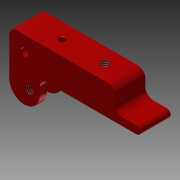
# Autodesk Inventor part: extruder_lever
Saved by Autodesk Inventor 2013 (Build 170138000, 138)
## iProperties
Created: 2015-02-21
Part Number: extruder_lever
Material: 一般
Document SubType Name: Modeling
Designer: Noa Izumi
Density: 1 g/cm^3
Author: Noa Izumi
Autodesk Inventor part; units mm, degrees
ref_plane "YZ Plane" through (0, 0, 0) normal (1, 0, 0) x (0, 1, 0)
ref_plane "XZ Plane" through (0, 0, 0) normal (0, 1, 0) x (-1, 0, 0)
ref_plane "XY Plane" through (0, 0, 0) normal (0, 0, 1) x (1, 0, 0)
sketch "草圖1" plane through (0, 0, 0) normal (0, 1, 0) x (-1, 0, 0)
  line L0 (0, 0) -> (42, 0)
  line L1 (42, 0) -> (42, 12)
  line L2 (42, 12) -> (0, 12)
  line L3 (0, 12) -> (0, 0)
  line L4 (0, 0) -> (-8.5, 0)
  line L5 (-10, 1.5) -> (-10, 1.5)
  line L6 (-8.5, 3) -> (0, 3)
  line L7 (0, 3) -> (0, 0)
  line L8 (30, 0) -> (42, 0)
  line L9 (42, 0) -> (42, -6)
  line L10 (36, -12) -> (36, -12)
  line L11 (30, -6) -> (30, 0)
  arc A0 (30, -6) -> (36, -12) centre (36, -6) ccw
  arc A1 (36, -12) -> (42, -6) centre (36, -6) ccw
  arc A2 (-8.5, 3) -> (-10, 1.5) centre (-8.5, 1.5) ccw
  arc A3 (-10, 1.5) -> (-8.5, 0) centre (-8.5, 1.5) ccw
  point P0 (-10, 3)
  point P1 (-10, 0)
  point P2 (42, -12)
  point P3 (30, -12)
  dimension "d0" = 42
  dimension "d2" = 10
  dimension "d3" = 3
  dimension "d4" = 12
  dimension "d6" = 12
  dimension "d7" = 12
  dimension "d8" = 6
  dimension "d9" = 1.5
  constraints: 24 end point, 9 point on line, 8 point on circle, 8 tangent, 6 parallel, 4 centre point, 3 horizontal, 3 perpendicular, 2 concentric
  measures "d0" distance of L1.end L2.end
  measures "d2" distance of point (-10, 3) L6.end
  measures "d3" distance of point (-10, 0) point (-10, 3)
  measures "d4" distance of point (42, -12) point (30, -12)
  measures "d6" distance of L0.end L1.end
  measures "d7" distance of L8.end point (42, -12)
  measures "d8" radius of A0
  measures "d9" radius of A2
extrude "擠出1" add sketch "草圖1" along normal blind 12
fillet "圓角1" radius 3 4 edges at (-42, 6, 12) (-30, 6, 0) (0, 6, 3) (0, 6, 12)
sketch "草圖2" plane through (0, 12, 0) normal (0, 1, 0) x (1, 0, 0)
  line L0 (-42, 6) -> (-42, -9) projected
  line L1 (-39, -12) -> (-3, -12) projected
  point P0 (0, 0)
  point P1 (-36, -6)
  dimension "d13" = 6
  dimension "d14" = 6
  measures "d13" distance from line of point (-36, -6) L1
  measures "d14" distance from line of L0 point (-36, -6)
hole "孔1" at (-36, 12, 6) direction (0, -1, 0) diameter 3 end through all counterbore diameter 7 counterbore depth 2
sketch "草圖3" plane through (8.5, 0, 0) normal (0, 0, -1) x (-1, 0, 0)
  line L0 (35.5, 12) -> (35.5, 0) projected
  line L1 (0, 0) -> (35.5, 0) projected
  line L2 (35.5, 9) -> (50.5, 9)
  line L3 (50.5, 9) -> (50.5, 3)
  line L4 (50.5, 3) -> (35.5, 3)
  line L5 (35.5, 3) -> (35.5, 9)
  point P0 (8.5, 0)
  dimension "d22" = 6
  dimension "d24" = 15
  dimension "d25" = 3
  constraints: 8 end point, 2 parallel, 1 horizontal, 1 perpendicular, 1 point on line
  measures "d22" distance of L4.end L2.start
  measures "d24" distance of L3.end L4.end
  measures "d25" distance between parallel lines of L1 L4
extrude "擠出2" cut sketch "草圖3" along normal blind 12
sketch "草圖4" plane through (0, 12, 0) normal (0, 1, 0) x (1, 0, 0)
  line L0 (-30, 3) -> (-30, 6) projected
  point P0 (0, 0)
  point P1 (-34, 6)
  dimension "d28" = 4
  measures "d28" distance from line of L0 point (-34, 6)
hole "孔2" at (-34, 12, -6) direction (0, -1, 0) diameter 3.242 end through all counterbore diameter 7.5 counterbore depth 2 thread size "M4x0.7" class "6H" standard "ANSI Metric M Profile"
sketch "草圖5" plane through (-39, 0, 12) normal (0, 0, 1) x (1, 0, 0)
  line L0 (-3, 12) -> (-3, 0) projected
  point P0 (39, 0)
  point P1 (12, 6)
  dimension "d36" = 15
  measures "d36" distance from line of L0 point (12, 6)
hole "孔3" at (-27, 6, 12) direction (0, 0, -1) diameter 2.5 end through all
chamfer "倒角1" distance 0.25 angle 45 2 edges at (-27, 7.25, 12) (-27, 7.25, 0)
sketch "草圖6" plane through (-39, 0, 12) normal (0, 0, 1) x (1, 0, 0)
  line L0 (-3, 12) -> (-3, 0) projected
  point P0 (39, 0)
  point P1 (29, 6)
  dimension "d47" = 32
  measures "d47" distance from line of point (29, 6) L0
hole "孔4" at (-10, 6, 12) direction (0, 0, -1) diameter 3.242 end through all thread size "M4x0.7" class "6H" standard "ANSI Metric M Profile"
